enz one two parts 4_v4 (Autodesk Fusion 360 design; units mm, degrees)
Autodesk Fusion 360 part; units mm, degrees
note: some values were not read from the file. Set by a fixed rule: which sketch regions a step uses.
sketch "base" plane through (0, 0, 0) normal (0, 0, 1) x (1, 0, 0)
  circle A0 centre (-21, 0.0874) radius 6.2
  circle A1 centre (-21, 0.0874) radius 7.1
  circle A2 centre (0, 0) radius 32.9
  circle A3 centre (0, 0) radius 7.1
  circle A4 centre (-21, 0.0874) radius 7.8
  circle A5 centre (-21, 0.0874) radius 6.8
  circle A6 centre (-14.911, -14.7874) radius 7.1
  circle A7 centre (-0.0874, -21) radius 7.1
  circle A8 centre (14.7874, -14.911) radius 7.1
  circle A9 centre (21, -0.0874) radius 7.1
  circle A10 centre (14.911, 14.7874) radius 7.1
  circle A11 centre (0.0874, 21) radius 7.1
  circle A12 centre (-14.7874, 14.911) radius 7.1
  point P0 (-21, 0.0874)
  dimension "d6" = 14.2
  dimension "d54" = 14.2
  dimension "d65" = 360
  dimension "d67" = 21
  dimension "d68" = 12.4
  dimension "d71" = 15.6
  dimension "d84" = 65.8
  dimension "d93" = 13.6
  constraint concentric A0 A1
  constraint coincident A2.centre A3.centre
  constraint coincident P0 A0.centre
  constraint concentric A1 A4
  constraint concentric A4 A5
  measures "d6" diameter of A1
  measures "d54" diameter of A3
  measures "d67" horizontal distance of P0 A2.centre
  measures "d68" diameter of A0
  measures "d71" diameter of A4
  measures "d84" diameter of A2
  measures "d93" diameter of A5
sketch "rim" plane through (0, 0, 0) normal (0, 1, 0) x (1, 0, 0)
  line L0 (32.9, -37.2) -> (32.9, -49.2)
  line L1 (31.9, -49.196) -> (32.9, -49.2)
  line L2 (32.9, -49.2) -> (37.25, -52.1593)
  line L3 (31.8966, -50.0514) -> (34.9952, -52.1593)
  line L4 (34.9952, -52.1593) -> (37.25, -52.1593)
  line L5 (31.9, -49.196) -> (32.9, -49.2)
  line L6 (31.9, -49.196) -> (31.9, -37.2)
  line L7 (31.9, -49.196) -> (31.8966, -50.0514)
  line L8 (32.9, -37.2) -> (31.9, -37.2)
  point P0 (32.9, -37.2)
  dimension "d26" = 37.2
  dimension "d27" = 32.9
  dimension "d29" = 12
  dimension "d63" = 37.25
  dimension "d75" = 34
  dimension "d101" = 31.9
  dimension "d103" = 1
  constraint coincident P0 L0.start
  constraint parallel L2 L3
  constraint horizontal L4
  constraint perpendicular L1 L7
  constraint perpendicular L6 L8
  constraint parallel L0 L6
  measures "d26" vertical distance of origin L0.start
  measures "d27" horizontal distance of P0 origin
  measures "d29" distance of P0 L0.end
  measures "d63" horizontal distance of L2.end origin
  measures "d75" angle of L2 L5
  measures "d101" horizontal distance of origin L1.start
  measures "d103" horizontal distance of L6.end P0
revolve "Revolve2" add sketch "rim" angle 360 about axis through (0, 0, 1.75) along (0, 0, 1) makes body 1
extrude "seat" add sketch "base" along normal blind 2 from surface at 36 contours A2 | A4 bodies 1
extrude "tubes" add sketch "base" along normal blind 40 separate body contours A5 makes body 2
extrude "base (1)" add sketch "base" along normal blind 2 contours A0 | A5 bodies 2
extrude "tubeRim" add sketch "base" along normal blind 2 from surface at 38 contours A1 | A4 bodies 2
sketch "washerMold" plane through (0, 0, 0) normal (0, 0, 1) x (1, 0, 0)
  circle A0 centre (0, 0) radius 37.25
  circle A1 centre (0, 0) radius 32.9
  circle A2 centre (0, 0) radius 32.15
  circle A3 centre (0, 0) radius 38
  dimension "d85" = 74.5
  dimension "d86" = 65.8
  dimension "d87" = 76
  dimension "d88" = 64.3
  constraint concentric A0 A1
  constraint concentric A0 A2
  constraint concentric A2 A3
  measures "d85" diameter of A0
  measures "d86" diameter of A1
  measures "d87" diameter of A3
  measures "d88" diameter of A2
extrude "Extrude12" add sketch "washerMold" along normal blind 5 separate body makes body 3 at (37.8112, -3.7836, 1.6667) makes body 4 at (32.8591, -1.6399, 3.3333)
extrude "Extrude13" add sketch "washerMold" along normal blind 2 contours A0 bodies 3 4
chamfer "Chamfer1" distance 0.3 angle 45 1 edges at (-30.6736, -11.8971, 2) on bodies 3
chamfer "Chamfer2" distance 0.3 angle 45 1 edges at (-34.7292, 13.4702, 2) on bodies 3
fillet "Fillet2" radius 1.5 1 edges at (-27.3398, 2.5464, 38) on bodies 2
fillet "Fillet3" radius 2.5 1 edges at (-29.7412, 11.5355, 38) on bodies 1
equation "d6 = bigTubeOutsideDiameter + tubeWallThickness + tubeDiameterPlay"
equation "submergedTubeHeight = 36 mm"
equation "capHeightAndOverhead = 12 mm"
equation "bigTubeOutsideDiameter = 12.4 mm"
equation "largeRimOutsideDiameter = 74.5 mm"
equation "baseRimOutsideDiameter = 65.8 mm"
equation "generalThickness = 2 mm"
equation "tubeWallThickness = 1.2 mm"
equation "d26 = submergedTubeHeight + tubeWallThickness"
equation "d27 = baseRimOutsideDiameter / 2"
equation "d29 = capHeightAndOverhead"
equation "d39 = submergedTubeHeight + 2 * tubeBottomThickness"
equation "d42 = submergedTubeHeight + tubeBottomThickness - generalThickness"
equation "d43 = generalThickness"
equation "d51 = tubeBottomThickness"
equation "d54 = bigTubeOutsideDiameter + tubeWallThickness + tubeDiameterPlay"
equation "smallTubeOutsideDiameter = 12.4 mm"
equation "d63 = largeRimOutsideDiameter / 2"
equation "d65 = 360.00 °"
equation "tubeBottomThickness = 2 mm"
equation "d68 = bigTubeOutsideDiameter"
equation "d71 = bigTubeOutsideDiameter + tubeWallThickness + tubeBottomThickness"
equation "d72 = submergedTubeHeight + tubeBottomThickness"
equation "d73 = tubeBottomThickness"
equation "d75 = 34 °"
equation "d84 = baseRimOutsideDiameter"
equation "d85 = largeRimOutsideDiameter"
equation "d86 = baseRimOutsideDiameter"
equation "d87 = largeRimOutsideDiameter + 1.5 mm"
equation "d88 = baseRimOutsideDiameter - 1.5 mm"
equation "d93 = bigTubeOutsideDiameter + tubeWallThickness"
equation "tubeDiameterPlay = 0.6 mm"
equation "d101 = baseRimOutsideDiameter / 2 - reolvedPartThickness"
equation "reolvedPartThickness = 1 mm"
equation "d103 = reolvedPartThickness"
named bodies: "holder", "tube", "washer mold"
